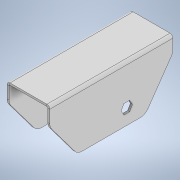
# Autodesk Inventor part: SP14V1 Pedal Derecho
Saved by Autodesk Inventor 2021.2 (Build 252289000, 289)
## iProperties
Created: 2026-06-16
Part Number: SP14V1 Pedal Derecho
Material: Generic
Document SubType Name: Sheet Metal
Designer: nelso
Density: 1 g/cm^3
Sheet Metal Rule: Default_mm
Appearance: Default
Mass: 129.601 g
Surface Area: 863.591 cm^2
Volume: 129.601 cm^3
Flat Pattern Width: 20 cm
Flat Pattern Length: 23.7633 cm
Flat Pattern Area: 475.266 cm^2
Sheet Metal Width: 200.000 mm
Sheet Metal Length: 237.633 mm
Sheet Metal Area: 47526.573 mm^2
Author: nelso
Autodesk Inventor part; units mm, degrees
ref_plane "YZ Plane" through (0, 0, 0) normal (1, 0, 0) x (0, 1, 0)
ref_plane "XZ Plane" through (0, 0, 0) normal (0, 1, 0) x (-1, 0, 0)
ref_plane "XY Plane" through (0, 0, 0) normal (0, 0, 1) x (1, 0, 0)
sketch "Sketch1" plane through (0, 0, 0) normal (0, 1, 0) x (-1, 0, 0)
  line L0 (-30, -100) -> (30, -100)
  line L1 (30, -100) -> (30, 100)
  line L2 (30, 100) -> (-30, 100)
  line L3 (-30, 100) -> (-30, -100)
  line L4 (-30, -100) -> (30, 100) construction
  line L5 (30, -100) -> (-30, 100) construction
  line L6 (30, 0) -> (30, 40)
  line L7 (30, 0) -> (30, -25)
  line L8 (-30, -100) -> (0, -100)
  line L9 (-30, -100) -> (30, -100)
  line L10 (30, -25) -> (30, -100)
  line L11 (30, 40) -> (40, 100)
  point P0 (0, 0)
  dimension "d0" = 60
  dimension "d1" = 200
  dimension "d2" = 40
  dimension "d3" = 25
  dimension "d5" = 60
  dimension "d6" = 70
  measures "d0" distance of L2.end L1.end
  measures "d1" distance of L1.end L0.end
  measures "d2" distance of L6.start L6.end
  measures "d3" distance of L6.start L7.end
  measures "d5" distance of L9.end L0.start
  measures "d6" distance of L11.end L2.end
extrude "Plate1" add sketch "Sketch1" along normal blind 3.2
sketch "Sketch2" plane through (31.516, -1.516, 100) normal (1, 0, 0) x (0, 1, 0)
  line L0 (0, -200) -> (0, 0)
  line L1 (0, 0) -> (-85.284, 0)
  line L2 (-85.284, 0) -> (-85.284, -200)
  line L3 (-85.284, -200) -> (0, -200)
  constraints: 6 end point, 1 horizontal, 1 perpendicular, 1 vertical
edge flange "Flange1" height 90 angle 90 thickness 3.2 bend radius 1.516 thickness toward (1, 0, 0) relief straight relief width 3.2 relief depth 1.6 corner gap 1.516 corner form 0 edges at (30, 0, 0) (-30, 0, 70) (-30, 0, 20) (-30, 0, -12.5) (-30, 0, -62.5) wall of the first edge with corners at (31.516, -1.516, -100) (31.516, -1.516, 100) (31.516, -86.8, 100) (31.516, -86.8, -100)
bend "Bend1"
corner "Corner1"
sketch "Sketch5" plane through (34.716, -86.8, 100) normal (1, 0, 0) x (0, 0, -1)
  line L0 (65.7624, 25) -> (70.3812, 33)
  line L1 (70.3812, 33) -> (79.6188, 33)
  line L2 (79.6188, 33) -> (84.2376, 25)
  line L3 (84.2376, 25) -> (79.6188, 17)
  line L4 (79.6188, 17) -> (70.3812, 17)
  line L5 (70.3812, 17) -> (65.7624, 25)
  line L6 (0, 90) -> (200, 90) projected
  line L7 (0, 90) -> (0, 65)
  line L8 (0, 0) -> (0, 85.284) projected
  line L9 (200, 0) -> (0, 0) projected
  line L10 (100, 0) -> (155, 0)
  line L11 (155, 0) -> (200, 60)
  line L12 (200, 0) -> (200, 85.284) projected
  line L13 (0, 65) -> (45, 0)
  line L14 (0, 0) -> (200, 0) projected
  point P0 (100, 86.8)
  point P1 (75, 25)
  dimension "d35" = 16
  dimension "d38" = 25
  dimension "d40" = 55
  dimension "d42" = 65
  dimension "d43" = 30
  dimension "d48" = 55
  dimension "d49" = 75
  constraints: 20 end point, 4 point on line, 1 midpoint, 13 other
  measures "d35" distance between parallel lines of L4 L1
  measures "d38" distance of L6.start L7.end
  measures "d40" distance of L10.start L10.end
  measures "d42" distance from line of L6 point (75, 25)
  measures "d43" distance of L11.end L6.end
  measures "d48" distance of L10.start L13.end
  measures "d49" distance from line of L8 point (75, 25)
extrude "Cut3" cut sketch "Sketch5" against normal through all
mirror "Mirror2" about plane through (0, 0, 0) normal (0, 0, 1) remove original yes
fillet "Corner Round2" radius 15 8 edges at (33.116, -26.8, 100) (-33.116, -26.8, 100) (33.116, -86.8, 55) (-33.116, -86.8, 55) (-33.116, -21.8, -100) (33.116, -21.8, -100) (-33.116, -86.8, -55) (33.116, -86.8, -55)
equation "\"d36\" = Thickness"
equation "\"d7\" = Thickness"
equation "\"d8\" = BendReliefWidth"
equation "\"d9\" = BendReliefDepth"
equation "\"d10\" = MinimumRemnant"
equation "\"d11\" = TransitionRadius"
equation "\"d14\" = BendRadius"
equation "\"d15\" = CornerReliefSize"
equation "\"d16\" = GapSize"
equation "\"d17\" = JacobiRadiusSize"
equation "\"BendReliefWidth\" = Thickness"
equation "\"BendReliefDepth\" = 0.5 * Thickness"
equation "\"CornerReliefSize\" = 4 * Thickness"
equation "\"MinimumRemnant\" = 2 * Thickness"
equation "\"TransitionRadius\" = BendRadius"
equation "\"JacobiRadiusSize\" = BendRadius"
equation "\"GapSize\" = Thickness"
equation "\"Thickness\" = 3.2"
equation "\"BendRadius\" = 1.516"
body "Solid1"
